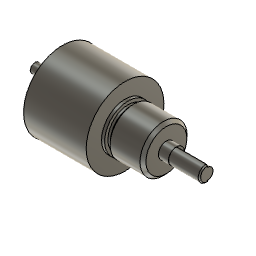
CALT P3015 v1 (Autodesk Fusion 360 design; units mm, degrees)
Autodesk Fusion 360 part; units mm, degrees
sketch "Sketch1" plane through (0, 0, 0) normal (0, 0, 1) x (1, 0, 0)
sketch "Sketch2" plane through (0, 0, 0) normal (0, 0, 1) x (1, 0, 0)
  line L0 (-1.5337, 1.9022) -> (1.5337, 1.9022)
  line L1 (1.5337, 1.9022) -> (1.5337, -1.9022)
  line L2 (1.5337, -1.9022) -> (-1.5337, -1.9022)
  line L3 (-1.5337, -1.9022) -> (-1.5337, 1.9022)
  line L4 (1.5337, 1.1527) -> (1.6853, 1.1527)
  line L5 (1.6853, 1.1527) -> (1.6853, -1.1241)
  line L6 (1.6853, -1.1241) -> (1.5337, -1.1241)
  line L7 (1.5337, -1.1241) -> (1.5337, 1.1527)
  line L8 (1.9529, 1.1527) -> (3.4161, 1.1527)
  line L9 (3.4161, 1.1527) -> (3.4161, -1.1241)
  line L10 (3.4161, -1.1241) -> (1.9529, -1.1241)
  line L11 (1.9529, -1.1241) -> (1.9529, 1.1527)
  line L12 (1.6853, 0.9939) -> (1.8102, 0.9939)
  line L13 (1.8102, 0.9939) -> (1.8102, -1.0259)
  line L14 (1.8102, -1.0259) -> (1.6853, -1.0259)
  line L15 (1.6853, -1.0259) -> (1.6853, 0.9939)
  line L16 (1.8102, 0.9939) -> (1.9529, 1.1527)
  line L17 (1.8102, -1.0259) -> (1.9529, -1.1241)
  line L18 (3.556, 0.3892) -> (4.0504, 0.3892)
  line L19 (4.0504, 0.3892) -> (4.0504, -0.3857)
  line L20 (4.0504, -0.3857) -> (3.556, -0.3857)
  line L21 (3.556, -0.3857) -> (3.556, 0.3892)
  line L22 (4.0504, 0.2799) -> (5.5052, 0.2799)
  line L23 (5.5052, 0.2799) -> (5.5052, -0.3857)
  line L24 (5.5052, -0.3857) -> (4.0504, -0.3857)
  line L25 (4.0504, -0.3857) -> (4.0504, 0.2799)
  line L26 (5.5052, 0.2799) -> (5.567, 0.2799)
  line L27 (5.567, 0.2799) -> (5.567, -0.3334)
  line L28 (5.567, -0.3334) -> (5.5052, -0.3334)
  line L29 (5.5052, -0.3334) -> (5.5052, 0.2799)
  line L30 (5.5052, -0.3857) -> (5.567, -0.3334)
  line L31 (3.556, -0.9998) -> (3.4161, -0.9998)
  line L32 (3.4161, -0.9998) -> (3.4161, 1.0016)
  line L33 (3.4161, 1.0016) -> (3.556, 1.0016)
  line L34 (3.556, 1.0016) -> (3.556, -0.9998)
  line L35 (3.4161, 1.1527) -> (3.556, 1.0016)
  line L36 (3.556, -0.9998) -> (3.4161, -1.1241)
  line L37 (-1.5337, 1.9022) -> (1.5337, -1.9022)
  line L38 (-1.5337, -1.9022) -> (1.5337, 1.9022)
  line L39 (0, 0) -> (5.567, 0)
  line L40 (-1.5337, 0) -> (0, 0)
  line L41 (3.557, -1.1241) -> (1.8102, -1.1241)
  line L42 (1.8102, -1.1241) -> (1.8102, 1.1506)
  line L43 (1.8102, 1.1506) -> (3.557, 1.1506)
  line L44 (3.557, 1.1506) -> (3.557, -1.1241)
  constraint horizontal L0
  constraint vertical L1
  constraint horizontal L2
  constraint vertical L3
  constraint horizontal L4
  constraint vertical L5
  constraint horizontal L6
  constraint vertical L7
  constraint coincident L1 L4.start
  constraint horizontal L8
  constraint vertical L9
  constraint horizontal L10
  constraint vertical L11
  constraint horizontal L12
  constraint vertical L13
  constraint horizontal L14
  constraint vertical L15
  constraint coincident L5 L12.start
  constraint horizontal L18
  constraint vertical L19
  constraint horizontal L20
  constraint vertical L21
  constraint horizontal L22
  constraint vertical L23
  constraint horizontal L24
  constraint vertical L25
  constraint coincident L19 L22.start
  constraint horizontal L26
  constraint vertical L27
  constraint horizontal L28
  constraint vertical L29
  constraint horizontal L31
  constraint vertical L32
  constraint horizontal L33
  constraint vertical L34
  constraint coincident L9 L32.end
  constraint midpoint L38 L39.start
  constraint midpoint L3 L40.start
  constraint coincident L27 L39.end
  constraint perpendicular L27 L39
  constraint coincident L37 L39.start
  constraint perpendicular L27 L40
  constraint horizontal L41
  constraint vertical L42
  constraint horizontal L43
  constraint vertical L44
revolve "Revolve1" add sketch "Sketch2" angle 360 about axis through (0, 0, 0) along (1, 0, 0) contours L3 L37 L40 | L0 L37 L38 | L1 L7 L38 L39 | L1 L4 L5 L7 L15 L39 | L5 L12 L13 L15 L39 L42 | L11 L13 L16 L39 L42 | L8 L9 L11 L32 L39 L43 | L9 L21 L32 L33 L34 L39 L44 | L9 L33 L35 | L18 L19 L21 L25 L34 L39 L44
revolve "Revolve2" add sketch "Sketch2" angle 360 about axis through (0, 0, 0) along (1, 0, 0) contours L19 L22 L23 L25 L29 L39 | L23 L26 L27 L29 L39
revolve "Revolve3" add sketch "Sketch2" angle 90 about axis through (0, 0, 0) along (1, 0, 0) second angle 90 contours L19 L23 L24 L25 L29 L39 | L23 L27 L28 L29 L39 | L23 L28 L30
scale "Scale1" factor 3.97782 about (-1.5337, 1.9022, 0) bodies 1
move_body "Move1" bodies 1 to x (1, 0, 0) y (0, 1, 0) z (0, 0, 1) at (1.5337, 5.6643, 0)
sketch "Sketch3" plane through (0, 0, 0) normal (1, 0, 0) x (0, 1, 0)
sketch "Sketch4" plane through (0, 0, 0) normal (1, 0, 0) x (0, 1, 0)
  line L0 (1.5289, 3.7323) -> (3.5974, 3.7323)
  circle A0 centre (2.5632, 3.7323) radius 0.9238
  circle A1 centre (-2.6368, 3.7323) radius 0.9238
  circle A2 centre (-0.0068, -4.5177) radius 0.9238
  constraint horizontal L0
  constraint midpoint L0 A0.centre
sketch "Sketch5" plane through (0, 0, 0) normal (0, 1, 0) x (1, 0, 0)
extrude "Extrude1" add sketch "Sketch4" against normal blind 2.7
